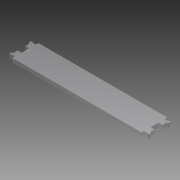
# Autodesk Inventor part: LeftPanel
Saved by Autodesk Inventor 2015 SP1 (Build 190203100, 203)
## iProperties
Created: 2015-01-22
Part Number: LeftPanel
Material: Acrylic, Clear
Document SubType Name: Modeling
Designer: Patrick
Density: 1.19 g/cm^3
Appearance: Transparent - Clear
Author: Patrick
Autodesk Inventor part; units mm, degrees
ref_plane "YZ Plane" through (0, 0, 0) normal (1, 0, 0) x (0, 1, 0)
ref_plane "XZ Plane" through (0, 0, 0) normal (0, 1, 0) x (-1, 0, 0)
ref_plane "XY Plane" through (0, 0, 0) normal (0, 0, 1) x (1, 0, 0)
sketch "Sketch1" plane through (0, 0, 0) normal (0, 0, 1) x (1, 0, 0)
  line L0 (-50, 10) -> (50, 10)
  line L1 (50, 10) -> (50, -10)
  line L2 (50, -10) -> (-50, -10)
  line L3 (-50, -10) -> (-50, 10)
  line L4 (-50, 10) -> (50, -10) construction
  line L5 (50, 10) -> (-50, -10) construction
  point P0 (0, 0)
  dimension "d0" = 100
  dimension "d1" = 20
  constraints: 12 end point, 2 midpoint, 2 parallel, 1 horizontal, 1 perpendicular
  measures "d0" distance of L1.end L2.end
  measures "d1" distance of L0.end L1.end
extrude "Extrusion1" add sketch "Sketch1" along normal blind 3
sketch "Sketch2" plane through (0, 0, 0) normal (0, 0, -1) x (-1, 0, 0)
  line L0 (-50, 8) -> (-53, 8)
  line L1 (-53, 8) -> (-53, 3)
  line L2 (-53, 3) -> (-50, 3)
  line L3 (-50, 3) -> (-50, 8)
  line L4 (-50, -8) -> (-53, -8)
  line L5 (-53, -8) -> (-53, -3)
  line L6 (-53, -3) -> (-50, -3)
  line L7 (-50, -3) -> (-50, -8)
  arc A0 (-53, 8.7) -> (-53, 6.3) centre (-53, 7.5) ccw
  arc A1 (-53, -6.3) -> (-53, -8.7) centre (-53, -7.5) ccw
  line L8 (-53, 8.7) -> (-53, 6.3)
  line L9 (-53, -6.3) -> (-53, -8.7)
  line L10 (-50, 10) -> (-50, -10) projected
  line L11 (50, 10) -> (-50, 10) projected
  line L12 (-50, -10) -> (50, -10) projected
  point P0 (0, 0)
  dimension "d15" = 3
  dimension "d16" = 5
  dimension "d17" = 5
  dimension "d18" = 1.2
  dimension "d19" = 1.2
  dimension "d20" = 0.5
  dimension "d21" = 0.5
  dimension "d22" = 2
  dimension "d23" = 2
  constraints: 20 end point, 4 parallel, 4 point on circle, 2 centre point, 2 collinear, 2 horizontal, 2 perpendicular, 2 point on line, 2 vertical
  measures "d15" distance of L3.start L1.end
  measures "d16" distance of L1.end L0.end
  measures "d17" distance of L4.end L5.end
  measures "d18" radius of A0
  measures "d19" radius of A1
  measures "d20" distance from line of L0 A0.centre
  measures "d21" distance from line of L4 A1.centre
  measures "d22" distance between parallel lines of L0 L11
  measures "d23" distance between parallel lines of L4 L12
extrude "Extrusion2" add sketch "Sketch2" against normal blind 3
mirror "Mirror1" about plane through (0, 0, 0) normal (1, 0, 0) of "Extrusion2"
equation "\"d17\" = d16"
equation "\"d23\" = d22"
body "Solid1"
